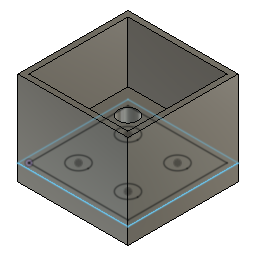
adaptor box final (Autodesk Fusion 360 design; units mm, degrees)
Autodesk Fusion 360 part; units mm, degrees
sketch "Sketch1" plane through (0, 0, 0) normal (0, 0, 1) x (1, 0, 0)
  line L0 (0, 0) -> (180, 0)
  line L1 (180, 0) -> (180, 180)
  line L2 (180, 180) -> (0, 180)
  line L3 (0, 180) -> (0, 0)
  line L4 (-10, -10) -> (190, -10)
  line L5 (190, -10) -> (190, 190)
  line L6 (190, 190) -> (-10, 190)
  line L7 (-10, 190) -> (-10, -10)
  circle A0 centre (45, 45) radius 17.5
  circle A1 centre (45, 135) radius 17.5
  circle A2 centre (135, 135) radius 17.5
  circle A3 centre (135, 45) radius 17.5
  dimension "d1" = 180
  dimension "d2" = 180
  dimension "d3" = 35
  dimension "d4" = 35
  dimension "d5" = 45
  dimension "d6" = 45
  dimension "d7" = 45
  dimension "d8" = 45
  dimension "d9" = 35
  dimension "d10" = 45
  dimension "d11" = 45
  dimension "d12" = 35
  dimension "d13" = 45
  dimension "d14" = 45
  constraint horizontal L0
  constraint vertical L1
  constraint horizontal L2
  constraint vertical L3
  constraint coincident L0.start L3.end
  constraint horizontal L4
  constraint vertical L5
  constraint horizontal L6
  constraint vertical L7
  measures "d1" distance of L0.start L2.end
  measures "d2" distance of L0.start L0.end
  measures "d3" diameter of A0
  measures "d4" diameter of A1
  measures "d5" distance of L2 A1.centre
  measures "d6" distance of L3 A1.centre
  measures "d7" distance of L0 A0.centre
  measures "d8" distance of L3 A0.centre
  measures "d9" diameter of A2
  measures "d10" distance of L2 A2.centre
  measures "d11" distance of L1 A2.centre
  measures "d12" diameter of A3
  measures "d13" distance of L1 A3.centre
  measures "d14" distance of L0 A3.centre
extrude "Extrude1" add sketch "Sketch1" along normal blind 140 contours L4 L5 L6 L7
extrude "Extrude2" add sketch "Sketch1" against normal blind 30 contours L0 L1 L2 L3 | L4 L5 L6 L7 | A0 | A1 | A2 | A3
extrude "Extrude3" add sketch "Sketch1" along normal blind 30 contours L0 L1 L2 L3
